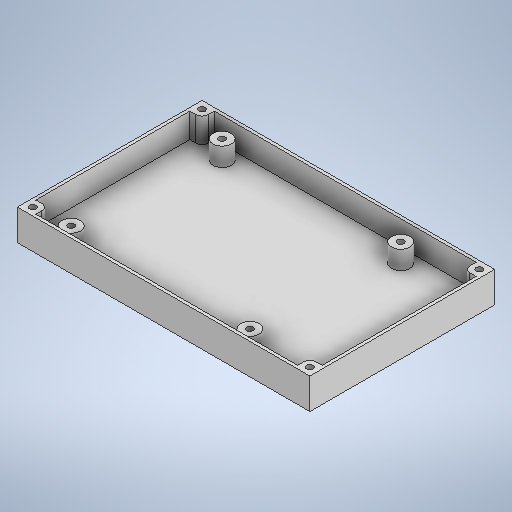
# Autodesk Inventor part: dol
Saved by Autodesk Inventor 2025 (Build 290162000, 162)
## iProperties
Created: 2024-12-16
Part Number: dol
Material: Ogólny
Document SubType Name: Modeling
Designer: Admin
Density: 1 g/cm^3
Appearance: Domyślna
Author: Admin
Autodesk Inventor part; units mm, degrees
ref_plane "YZ Plane" through (0, 0, 0) normal (1, 0, 0) x (0, 1, 0)
ref_plane "XZ Plane" through (0, 0, 0) normal (0, 1, 0) x (-1, 0, 0)
ref_plane "XY Plane" through (0, 0, 0) normal (0, 0, 1) x (1, 0, 0)
sketch "Szkic1" plane through (0, 0, 0) normal (0, 1, 0) x (-1, 0, 0)
  line L0 (0, 0) -> (90, 0)
  line L1 (90, 0) -> (90, -60)
  line L2 (90, -60) -> (0, -60)
  line L3 (0, -60) -> (0, 0)
  dimension "d0" = 90
  dimension "d1" = 60
  constraints: 8 end point, 2 perpendicular, 1 horizontal, 1 vertical
  measures "d0" distance of L0.start L0.end
  measures "d1" distance of L0.end L1.end
extrude "Wyciągnięcie proste1" add sketch "Szkic1" along normal blind 2
sketch "Szkic10" plane through (0, 2, 0) normal (0, 1, 0) x (1, 0, 0)
  circle A0 centre (-83, 54.5) radius 3
  circle A1 centre (-25, 54.5) radius 3
  circle A2 centre (-25, 5.5) radius 3
  circle A3 centre (-83, 5.5) radius 3
  point P0 (0, 0)
  dimension "d21" = 6
  dimension "d22" = 6
  dimension "d23" = 6
  dimension "d24" = 6
  constraints: 4 centre point, 4 coincident
  measures "d21" diameter of A0
  measures "d22" diameter of A1
  measures "d23" diameter of A2
  measures "d24" diameter of A3
extrude "Wyciągnięcie proste4" add sketch "Szkic10" along normal blind 6
sketch "Szkic11" plane through (-83, 8, -54.5) normal (0, 1, 0) x (1, 0, 0)
  circle A0 centre (0, 0) radius 3 projected
  point P0 (83, -54.5)
  constraints: 1 coincident
hole "Otwór1" at (-83, 8, -54.5) direction (0, -1, 0) diameter 2.1129 depth 4 tip angle 118 counterbore diameter 2.7 counterbore depth 0 thread size "M2.6x0.45" class "6H" standard "ISO Metric profile"
sketch "Szkic12" plane through (-83, 8, -5.5) normal (0, 1, 0) x (1, 0, 0)
  circle A0 centre (0, 0) radius 3 projected
  point P0 (83, -5.5)
  constraints: 1 coincident
hole "Otwór2" at (-83, 8, -5.5) direction (0, -1, 0) diameter 2.1129 depth 4 tip angle 118 counterbore diameter 2.7 counterbore depth 0 thread size "M2.6x0.45" class "6H" standard "ISO Metric profile"
sketch "Szkic13" plane through (-25, 8, -54.5) normal (0, 1, 0) x (1, 0, 0)
  point P0 (25, -54.5)
  point P1 (0, 0)
  point P2 (0, 0)
  constraints: 1 coincident
hole "Otwór3" at (-25, 8, -54.5) direction (0, -1, 0) diameter 2.1129 depth 4 tip angle 118 counterbore diameter 2.7 counterbore depth 0 thread size "M2.6x0.45" class "6H" standard "ISO Metric profile"
sketch "Szkic14" plane through (-25, 8, -5.5) normal (0, 1, 0) x (1, 0, 0)
  point P0 (25, -5.5)
  point P1 (0, 0)
  point P2 (0, 0)
  constraints: 1 coincident
hole "Otwór4" at (-25, 8, -5.5) direction (0, -1, 0) diameter 2.1129 depth 4 tip angle 118 counterbore diameter 2.7 counterbore depth 0 thread size "M2.6x0.45" class "6H" standard "ISO Metric profile"
sketch "Szkic15" plane through (-90, 0, -60) normal (-1, 0, 0) x (0, 0, 1)
  line L0 (0, 0) -> (60, 0)
  line L1 (60, 0) -> (60, 2)
  line L2 (60, 2) -> (0, 2)
  line L3 (0, 2) -> (0, 0)
  constraints: 8 end point, 2 parallel, 1 horizontal, 1 perpendicular
extrude "Wyciągnięcie proste5" add sketch "Szkic15" along normal blind 5
sketch "Szkic16" plane through (0, 2, 0) normal (0, 1, 0) x (1, 0, 0)
  line L0 (0, 60) -> (-95, 60) projected
  line L1 (-95, 60) -> (-95, 0) projected
  line L2 (-94, 60) -> (-95, 60)
  line L3 (-95, 60) -> (-95, 0)
  line L4 (-95, 0) -> (-94, 0)
  line L5 (-94, 0) -> (-94, 60)
  line L6 (-95, 1) -> (0, 1)
  line L7 (0, 1) -> (0, 0)
  line L8 (0, 0) -> (-95, 0)
  line L9 (-95, 0) -> (-95, 1)
  line L10 (-1, 0) -> (0, 0)
  line L11 (0, 0) -> (0, 60)
  line L12 (0, 60) -> (-1, 60)
  line L13 (-1, 60) -> (-1, 0)
  line L14 (-1, 59) -> (-95, 59)
  line L15 (-95, 59) -> (-95, 60)
  line L16 (-95, 60) -> (-1, 60)
  line L17 (-1, 60) -> (-1, 59)
  point P0 (-94, 59)
  point P1 (-1, 1)
  point P2 (-94, 1)
  constraints: 32 end point, 8 parallel, 6 point on line, 4 horizontal, 4 perpendicular
extrude "Wyciągnięcie proste6" add sketch "Szkic16" along normal blind 8 contours L11 L6 L13 L0 | L13 L14 L5 L0 | L7 L8 L13 L6 | L5 L14 L1 L0 | L13 L8 L5 L6 | L5 L6 L1 L14 | L5 L4 L1 L6
sketch "Szkic21" plane through (0, 2, 0) normal (0, 1, 0) x (1, 0, 0)
  line L0 (-1, 59) -> (-1, 1) projected
  line L1 (-94, 1) -> (-1, 1) projected
  line L2 (-1, 5) -> (-5, 5)
  line L3 (-5, 5) -> (-5, 1)
  line L4 (-5, 1) -> (-1, 1)
  line L5 (-1, 1) -> (-1, 5)
  point P0 (0, 0)
  dimension "d61" = 4
  constraints: 8 end point, 2 parallel, 2 point on line, 1 horizontal, 1 perpendicular
  measures "d61" distance of L4.end L3.end
extrude "Wyciągnięcie proste8" add sketch "Szkic21" along normal blind 8
sketch "Szkic22" plane through (0, 2, 0) normal (0, 1, 0) x (1, 0, 0)
  line L0 (-1, 59) -> (-1, 5) projected
  line L1 (-1, 55) -> (-5, 55)
  line L2 (-5, 55) -> (-5, 59)
  line L3 (-5, 59) -> (-1, 59)
  line L4 (-1, 59) -> (-1, 55)
  line L5 (-94, 1) -> (-94, 59) projected
  line L6 (-1, 59) -> (-94, 59) projected
  line L7 (-94, 55) -> (-90, 55)
  line L8 (-90, 55) -> (-90, 59)
  line L9 (-90, 59) -> (-94, 59)
  line L10 (-94, 59) -> (-94, 55)
  line L11 (-94, 1) -> (-5, 1) projected
  line L12 (-94, 5) -> (-90, 5)
  line L13 (-90, 5) -> (-90, 1)
  line L14 (-90, 1) -> (-94, 1)
  line L15 (-94, 1) -> (-94, 5)
  point P0 (0, 0)
  dimension "d64" = 4
  dimension "d65" = 4
  constraints: 24 end point, 6 parallel, 6 point on line, 3 horizontal, 3 perpendicular
  measures "d64" distance of L2.end L3.end
  measures "d65" distance of L9.end L8.end
extrude "Wyciągnięcie proste9" add sketch "Szkic22" along normal blind 8
fillet "Zaokrąglenie1" radius 2 4 edges at (-90, 6, -55) (-5, 6, -55) (-90, 6, -5) (-5, 6, -5)
sketch "Szkic23" plane through (0, 10, 0) normal (0, 1, 0) x (1, 0, 0)
  point P0 (0, 0)
  point P1 (-2.5, 2.5)
  point P2 (-92.5, 2.5)
  point P3 (-92.5, 57.5)
  point P4 (-2.5, 57.5)
hole "Otwór5" at (-2.5, 10, -2.5) at (-92.5, 10, -2.5) at (-92.5, 10, -57.5) at (-2.5, 10, -57.5) direction (0, -1, 0) diameter 2.1129 depth 4 tip angle 118 counterbore diameter 2.7 counterbore depth 0 thread size "M2.6x0.45" class "6H" standard "ISO Metric profile"
equation "\"d25\" = d22"
